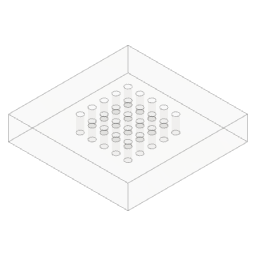
parametricBitHolderBlock (Autodesk Fusion 360 design; units mm, degrees)
Autodesk Fusion 360 part; units mm, degrees
sketch "Sketch1" plane through (0, 0, 0) normal (0, 0, 1) x (1, 0, 0) in component "base"
  line L0 (0, 0) -> (127, 0)
  line L1 (127, 0) -> (127, 127)
  line L2 (127, 127) -> (0, 127)
  line L3 (0, 127) -> (0, 0)
  dimension "d1" = 127
  dimension "d2" = 127
  constraint horizontal L0
  constraint vertical L1
  constraint horizontal L2
  constraint vertical L3
  constraint coincident L0.start L3.end
  measures "d1" distance of L1.end L2.end
  measures "d2" distance of L0.end L1.end
extrude "Extrude1" add sketch "Sketch1" along normal blind 25.4 in component "base"
hole "Hole1" at (38.1, 38.1, 25.4) direction (0, 0, -1) diameter 6.35 depth 16.9333 tip angle 180 in component "base"
pattern_linear "R-Pattern1" count 5 spacing 12.7 along (1, 0, 0) count 5 spacing 12.7 along (0, 1, 0) of "Hole1" in component "base"
sketch "Sketch1 (2)" plane through (0, 0, 0) normal (0, 0, 1) x (1, 0, 0) in component "projectedSketch"
  circle A0 centre (88.9, 50.8) radius 3.175
  circle A1 centre (76.2, 50.8) radius 3.175
  circle A2 centre (63.5, 50.8) radius 3.175
  circle A3 centre (50.8, 50.8) radius 3.175
  circle A4 centre (38.1, 50.8) radius 3.175
  circle A5 centre (88.9, 38.1) radius 3.175
  circle A6 centre (76.2, 38.1) radius 3.175
  circle A7 centre (63.5, 38.1) radius 3.175
  circle A8 centre (50.8, 38.1) radius 3.175
  circle A9 centre (38.1, 38.1) radius 3.175
  line L0 (0, 127) -> (0, 0)
  line L1 (0, 0) -> (127, 0)
  line L2 (127, 0) -> (127, 127)
  line L3 (127, 127) -> (0, 127)
  circle A10 centre (88.9, 88.9) radius 3.175
  circle A11 centre (76.2, 88.9) radius 3.175
  circle A12 centre (63.5, 88.9) radius 3.175
  circle A13 centre (50.8, 88.9) radius 3.175
  circle A14 centre (38.1, 88.9) radius 3.175
  circle A15 centre (88.9, 76.2) radius 3.175
  circle A16 centre (76.2, 76.2) radius 3.175
  circle A17 centre (63.5, 76.2) radius 3.175
  circle A18 centre (50.8, 76.2) radius 3.175
  circle A19 centre (38.1, 76.2) radius 3.175
  circle A20 centre (88.9, 63.5) radius 3.175
  circle A21 centre (76.2, 63.5) radius 3.175
  circle A22 centre (63.5, 63.5) radius 3.175
  circle A23 centre (50.8, 63.5) radius 3.175
  circle A24 centre (38.1, 63.5) radius 3.175
component "base" placed x (1, 0, 0) y (0, 1, 0) z (0, 0, 1) at (0, 0, 0)
component "projectedSketch" placed x (1, 0, 0) y (0, 1, 0) z (0, 0, 1) at (0, 0, 0)
equation "d1 = length"
equation "d2 = width"
equation "length = 5 in"
equation "width = 5 in"
equation "thickness = 1 in"
equation "bitSize1 = 0.25 in"
equation "bitSize2 = 0.125 in"
equation "d8 = thickness"
equation "d10 = bitDepth"
equation "d11 = bitSize1"
equation "d13 = yEdge"
equation "d14 = xEdge"
equation "bitDepth = 2 * thickness / 3"
equation "xSpacing = 0.5 in"
equation "ySpacing = 0.5 in"
equation "d18 = xQuantity"
equation "d19 = yQuantity"
equation "d20 = xSpacing"
equation "d21 = ySpacing"
equation "xQuantity = 5"
equation "yQuantity = 5"
equation "xEdge = ( length - ( xSpacing * ( xQuantity - 1 ) ) ) / 2"
equation "yEdge = ( width - ( ySpacing * ( yQuantity - 1 ) ) ) / 2"
